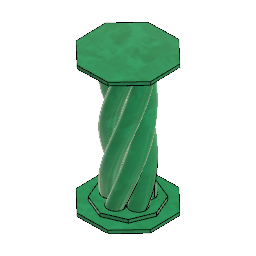
column (Autodesk Fusion 360 design; units mm, degrees)
Autodesk Fusion 360 part; units mm, degrees
sketch "Base big octogon" plane through (0, 0, 0) normal (0, 0, 1) x (1, 0, 0)
  line L0 (35.2747, -13.8156) -> (34.7121, 15.1739)
  line L1 (34.7121, 15.1739) -> (13.8156, 35.2747)
  line L2 (13.8156, 35.2747) -> (-15.1739, 34.7121)
  line L3 (-15.1739, 34.7121) -> (-35.2747, 13.8156)
  line L4 (-35.2747, 13.8156) -> (-34.7121, -15.1739)
  line L5 (-34.7121, -15.1739) -> (-13.8156, -35.2747)
  line L6 (-13.8156, -35.2747) -> (15.1739, -34.7121)
  line L7 (15.1739, -34.7121) -> (35.2747, -13.8156)
  dimension "d1" = 35
  measures "d1" distance of origin L7
extrude "Extrude1" add sketch "Base big octogon" along normal blind 3 makes body 1
sketch "Base small octogon" plane through (0, 0, 3) normal (0, 0, 1) x (-1, 0, 0)
  line L0 (-15.1739, 34.7121) -> (-35.2747, 13.8156)
  line L1 (-35.2747, 13.8156) -> (-34.7121, -15.1739)
  line L2 (-34.7121, -15.1739) -> (-13.8156, -35.2747)
  line L3 (-13.8156, -35.2747) -> (15.1739, -34.7121)
  line L4 (15.1739, -34.7121) -> (35.2747, -13.8156)
  line L5 (35.2747, -13.8156) -> (34.7121, 15.1739)
  line L6 (34.7121, 15.1739) -> (13.8156, 35.2747)
  line L7 (13.8156, 35.2747) -> (-15.1739, 34.7121)
  line L8 (-27.0589, -0.2164) -> (-18.9806, -19.2866)
  line L9 (-18.9806, -19.2866) -> (0.2164, -27.0589)
  line L10 (0.2164, -27.0589) -> (19.2866, -18.9806)
  line L11 (19.2866, -18.9806) -> (27.0589, 0.2164)
  line L12 (27.0589, 0.2164) -> (18.9806, 19.2866)
  line L13 (18.9806, 19.2866) -> (-0.2164, 27.0589)
  line L14 (-0.2164, 27.0589) -> (-19.2866, 18.9806)
  line L15 (-19.2866, 18.9806) -> (-27.0589, -0.2164)
  dimension "d4" = 25
  measures "d4" distance of origin L15
extrude "Extrude2" add sketch "Base small octogon" along normal blind 3 contours L8 L9 L10 L11 L12 L13 L14 L15 bodies 1
ref_plane "WorkPlane1" through (0, 0, 120) normal (0, 0, 1) x (1, 0, 0)
sketch "Top small octogon" plane through (0, 0, 120) normal (0, 0, 1) x (1, 0, 0)
  line L0 (27.0543, 0.5446) -> (18.7452, 19.5154)
  line L1 (18.7452, 19.5154) -> (-0.5446, 27.0543)
  line L2 (-0.5446, 27.0543) -> (-19.5154, 18.7452)
  line L3 (-19.5154, 18.7452) -> (-27.0543, -0.5446)
  line L4 (-27.0543, -0.5446) -> (-18.7452, -19.5154)
  line L5 (-18.7452, -19.5154) -> (0.5446, -27.0543)
  line L6 (0.5446, -27.0543) -> (19.5154, -18.7452)
  line L7 (19.5154, -18.7452) -> (27.0543, 0.5446)
  dimension "d8" = 25
  measures "d8" distance of origin L7
extrude "Extrude3" add sketch "Top small octogon" along normal mid plane 6 separate body makes body 2
sketch "Top big octogon" plane through (0, 0, 123) normal (0, 0, 1) x (-1, 0, 0)
  line L0 (-19.5154, 18.7452) -> (-27.0543, -0.5446)
  line L1 (-27.0543, -0.5446) -> (-18.7452, -19.5154)
  line L2 (-18.7452, -19.5154) -> (0.5446, -27.0543)
  line L3 (0.5446, -27.0543) -> (19.5154, -18.7452)
  line L4 (19.5154, -18.7452) -> (27.0543, 0.5446)
  line L5 (27.0543, 0.5446) -> (18.7452, 19.5154)
  line L6 (18.7452, 19.5154) -> (-0.5446, 27.0543)
  line L7 (-0.5446, 27.0543) -> (-19.5154, 18.7452)
  line L8 (-34.6202, -15.3823) -> (-13.6032, -35.3572)
  line L9 (-13.6032, -35.3572) -> (15.3823, -34.6202)
  line L10 (15.3823, -34.6202) -> (35.3572, -13.6032)
  line L11 (35.3572, -13.6032) -> (34.6202, 15.3823)
  line L12 (34.6202, 15.3823) -> (13.6032, 35.3572)
  line L13 (13.6032, 35.3572) -> (-15.3823, 34.6202)
  line L14 (-15.3823, 34.6202) -> (-35.3572, 13.6032)
  line L15 (-35.3572, 13.6032) -> (-34.6202, -15.3823)
  dimension "d11" = 35
  measures "d11" distance of origin L15
extrude "Extrude4" add sketch "Top big octogon" along normal blind 3 separate body makes body 3
sketch "Columns" plane through (0, 0, 6) normal (0, 0, 1) x (-1, 0, 0)
  line L0 (-19.2866, 18.9806) -> (-27.0589, -0.2164)
  line L1 (-27.0589, -0.2164) -> (-18.9806, -19.2866)
  line L2 (-18.9806, -19.2866) -> (0.2164, -27.0589)
  line L3 (0.2164, -27.0589) -> (19.2866, -18.9806)
  line L4 (19.2866, -18.9806) -> (27.0589, 0.2164)
  line L5 (27.0589, 0.2164) -> (18.9806, 19.2866)
  line L6 (18.9806, 19.2866) -> (-0.2164, 27.0589)
  line L7 (-0.2164, 27.0589) -> (-19.2866, 18.9806)
  circle A0 centre (8.4273, -9.795) radius 7.5
  circle A1 centre (11.9198, 4.988) radius 7.5
  circle A2 centre (-1.0604, 12.8778) radius 7.5
  circle A3 centre (-12.5752, 2.9709) radius 7.5
  circle A4 centre (-6.7115, -11.0416) radius 7.5
  dimension "d14" = 15
  dimension "d16" = 360
  measures "d14" diameter of A0
sketch "Vertical line" plane through (0, 0, 0) normal (0, 1, 0) x (1, 0, 0)
  line L0 (0, -6) -> (0, -126)
  dimension "d17" = 120
  constraint vertical L0
  measures "d17" distance of L0.start L0.end
sweep "Sweep1" add twist angle 180 profiles "Columns" path "Vertical line" along L0 for 0.925 of its length starting at (0, 0, 6) heading (0, 0, 1) section 1 contours A0 | A1 | A2 | A3 | A4 bodies 1 3 2
extrude "Extrude5" add 1 faces at (-0.1815, 9.0181, 123) along direction (0, 0, 1) blind 3 on bodies 1 bodies 1 3
named bodies: "Column"
